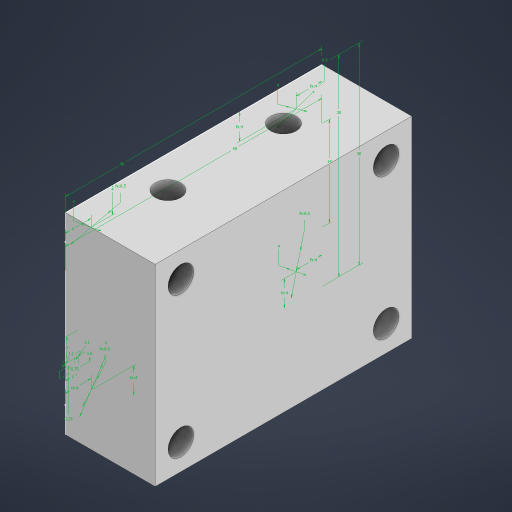
# Autodesk Inventor part: LRT_Face
Saved by Autodesk Inventor 2024.2 (Build 282272000, 272)
## iProperties
Created: 2024-09-29
Part Number: LRT_Face
Material: Generic
Document SubType Name: Modeling
Designer: jerem
Density: 1 g/cm^3
Appearance: Default
Author: jerem
Autodesk Inventor part; units mm, degrees
ref_plane "YZ Plane" through (0, 0, 0) normal (1, 0, 0) x (0, 1, 0)
ref_plane "XZ Plane" through (0, 0, 0) normal (0, 1, 0) x (-1, 0, 0)
ref_plane "XY Plane" through (0, 0, 0) normal (0, 0, 1) x (1, 0, 0)
sketch "Sketch1" plane through (0, 0, 0) normal (1, 0, 0) x (0, 1, 0)
  line L0 (-15, -20) -> (15, -20)
  line L1 (15, -20) -> (15, 20)
  line L2 (15, 20) -> (-15, 20)
  line L3 (-15, 20) -> (-15, -20)
  line L4 (-15, -20) -> (15, 20) construction
  line L5 (15, -20) -> (-15, 20) construction
  line L6 (-7, -20) -> (7, -20)
  line L7 (7, -20) -> (7, 20)
  line L8 (7, 20) -> (-7, 20)
  line L9 (-7, 20) -> (-7, -20)
  line L10 (7, -20) -> (5.4606, -20)
  arc A0 (-5.3073, 19.4579) -> (-4.85, 20) centre (-5.4, 20) ccw
  arc A1 (-4.85, 18) -> (-5.3073, 18.5421) centre (-5.4, 18) ccw
  line L11 (-5.4, 20) -> (-5.4, 18) construction
  line L12 (-6, 19.1286) -> (-6, 18.8714)
  line L13 (-5.7921, 19.375) -> (-5.3073, 19.4579)
  line L14 (-5.3073, 18.5421) -> (-5.7921, 18.625)
  arc A2 (-5.7921, 19.375) -> (-6, 19.1286) centre (-5.75, 19.1286) ccw
  arc A3 (-6, 18.8714) -> (-5.7921, 18.625) centre (-5.75, 18.8714) ccw
  line L15 (-5.4, 18) -> (-4.85, 18) construction
  line L16 (-6, 19) -> (-5.4, 19) construction
  line L17 (-4.85, 18) -> (-1.85, 18)
  line L18 (-1.85, 18) -> (-1.85, 20)
  line L19 (7, -20) -> (-7, 20) construction
  line L20 (7, 20) -> (-7, -20) construction
  line L21 (7, 20) -> (15, 20)
  line L22 (15, 20) -> (15, -20)
  line L23 (15, -20) -> (7, -20)
  line L24 (-7, 20) -> (-15, 20)
  line L25 (-15, 20) -> (-15, -20)
  line L26 (-15, -20) -> (-7, -20)
  circle A4 centre (11, 16) radius 2
  circle A5 centre (11, -16) radius 2
  circle A6 centre (-11, 16) radius 2
  circle A7 centre (-11, -16) radius 2
  circle A8 centre (11, -16) radius 3.25
  circle A9 centre (11, 16) radius 3.25
  circle A10 centre (-11, 16) radius 3.25
  circle A11 centre (-11, -16) radius 3.25
  point P0 (0, 0)
  point P1 (0, 0)
  point P2 (5.4606, -20)
  point P3 (11, 20)
  point P4 (-11, 20)
  dimension "d0" = 40
  dimension "d1" = 30
  dimension "d12" = 14
  dimension "d13" = 1.1
  dimension "d14" = 1.6
  dimension "d15" = 1.1
  dimension "d16" = 2
  dimension "d17" = 1
  dimension "d18" = 0.25
  dimension "d19" = 0.75
  dimension "d20" = 3
  dimension "d21" = 40
  dimension "d22" = 30
  dimension "d23" = 4
  dimension "d24" = 4
  dimension "d25" = 4
  dimension "d26" = 4
  dimension "d27" = 4
  dimension "d28" = 4
  dimension "d29" = 4
  dimension "d30" = 4
  dimension "d31" = 4
  dimension "d32" = 4
  dimension "d33" = 4
  dimension "d34" = 4
  dimension "d37" = 6.5
  dimension "d38" = 6.5
  dimension "d39" = 6.5
  dimension "d40" = 6.5
  constraints: 54 end point, 12 centre point, 8 point on circle, 7 midpoint, 7 perpendicular, 6 coincident, 6 horizontal, 6 point on line, 6 tangent, 4 parallel, 2 vertical, 1 collinear, 1 equal radius
  measures "d0" distance of L0.end L1.end
  measures "d1" distance of L0.start L0.end
  measures "d12" distance between parallel lines of L9 L7
  measures "d13" diameter of A0
  measures "d14" distance of L8.end L11.start
  measures "d15" diameter of A1
  measures "d16" distance of L11.end L11.start
  measures "d17" distance between parallel lines of L9 L12
  measures "d18" radius of A2
  measures "d19" distance of L14.end L13.start
  measures "d20" distance of L17.start L17.end
  measures "d21" distance of L19.start L21.start
  measures "d22" distance between parallel lines of L25 L22
  measures "d23" diameter of A4
  measures "d24" diameter of A5
  measures "d25" distance from line of L22 A4.centre
  measures "d26" distance of point (11, 20) A4.centre
  measures "d27" distance from line of L23 A5.centre
  measures "d28" diameter of A6
  measures "d29" diameter of A7
  measures "d30" distance from line of L26 A7.centre
  measures "d31" distance from line of L25 A7.centre
  measures "d32" distance from line of L25 A6.centre
  measures "d33" distance of point (-11, 20) A6.centre
  measures "d34" distance from line of L22 A5.centre
  measures "d37" diameter of A8
  measures "d38" diameter of A11
  measures "d39" diameter of A10
  measures "d40" diameter of A9
extrude "Extrusion1" add sketch "Sketch1" along normal blind 14 contours L3 L2 L9 L0 | L9 L2 A0 L13 A2 L12 A3 L14 A1 L17 L18 L7 L0 | L7 L2 L1 L0 | L2 L18 L17 A1 L14 A3 L12 A2 L13 A0 | A4 | A5 | A6 | A7 | A8 | A9 | A10 | A11
sketch "Sketch2" plane through (0, 15, 20) normal (0, 1, 0) x (1, 0, 0)
  line L0 (0, 40) -> (0, 0) construction
  line L1 (0, 11) -> (5, 11) construction
  line L2 (0, 29) -> (5, 29) construction
  circle A0 centre (5, 11) radius 2
  circle A1 centre (5, 29) radius 2
  line L3 (0, 0) -> (14, 0) projected
  point P0 (0, 20)
  dimension "d4" = 5
  dimension "d5" = 5
  dimension "d6" = 4
  dimension "d7" = 4
  dimension "d8" = 18
  dimension "d9" = 11
  constraints: 4 end point, 2 centre point, 2 coincident, 2 point on line, 1 horizontal, 1 perpendicular
  measures "d4" distance of L1.start L1.end
  measures "d5" distance of L2.start L2.end
  measures "d6" diameter of A0
  measures "d7" diameter of A1
  measures "d8" distance between parallel lines of L2 L1
  measures "d9" distance from line of L3 L1.end
extrude "Extrusion2" cut sketch "Sketch2" against normal blind 3
mirror "Mirror1" about plane through (0, 0, 0) normal (0, 1, 0) of "Extrusion2"
extrude "Extrusion3" cut sketch "Sketch1" along normal through all contours A4 | A5 | A6 | A7
extrude "Extrusion4" cut sketch "Sketch1" along normal blind 5 contours A8 | A9 | A10 | A11
equation "\"d27\" = d26"
equation "\"d30\" = d27"
equation "\"d31\" = d25"
equation "\"d32\" = d23"
equation "\"d33\" = d26"
equation "\"d34\" = d23"
equation "\"d38\" = d37"
equation "\"d39\" = d37"
equation "\"d40\" = d37"
equation "\"d5\" = d4"
body "Solid1"
